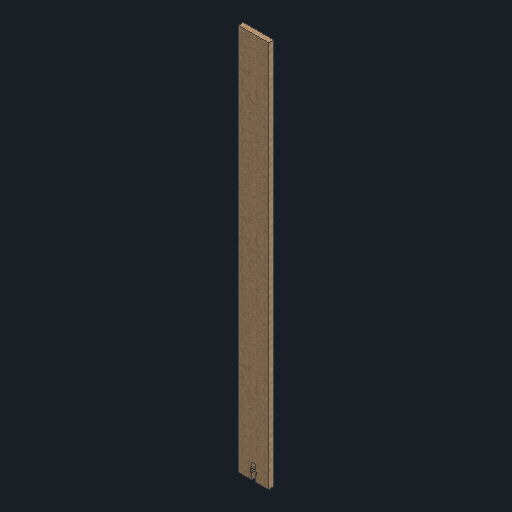
# Autodesk Inventor part: Reed_Rail
Saved by Autodesk Inventor 2024.1 (Build 281209000, 209)
## iProperties
Created: 2023-08-05
Part Number: Reed_Rail
Material: MDF Medium Density Fiberboard
Document SubType Name: Modeling
Designer: jaege
Density: 0.8 g/cm^3
Appearance: Cardboard - Corrugated
Author: jaege
Autodesk Inventor part; units mm, degrees
ref_plane "YZ Plane" through (0, 0, 0) normal (1, 0, 0) x (0, 1, 0)
ref_plane "XZ Plane" through (0, 0, 0) normal (0, 1, 0) x (-1, 0, 0)
ref_plane "XY Plane" through (0, 0, 0) normal (0, 0, 1) x (1, 0, 0)
sketch "Sketch1" plane through (0, 0, 0) normal (0, 0, 1) x (1, 0, 0)
  line L0 (-7, 315) -> (1, 315) projected
  line L1 (-7, 311) -> (-7, 315) projected
  line L2 (1, 311) -> (-7, 311) projected
  line L3 (1, 311) -> (1, 315) projected
  line L4 (-15, 311) -> (9, 311)
  line L5 (9, 311) -> (9, 4)
  line L6 (9, 4) -> (-15, 4)
  line L7 (-15, 4) -> (-15, 311)
  line L8 (-4.5, 4) -> (-1.5, 4)
  line L9 (-1.5, 4) -> (-1.5, 16)
  line L10 (-1.5, 16) -> (-4.5, 16)
  line L11 (-4.5, 16) -> (-4.5, 4)
  line L12 (-5.7, 11.2) -> (-0.3, 11.2)
  line L13 (-0.3, 11.2) -> (-0.3, 8.8)
  line L14 (-0.3, 8.8) -> (-5.7, 8.8)
  line L15 (-5.7, 8.8) -> (-5.7, 11.2)
  point P0 (-3, 311)
  point P1 (-3, 311)
  point P2 (-3, 4)
  point P3 (-3, 4)
  point P4 (-5.7, 10)
  point P5 (-4.5, 10)
  point P6 (-3, 11.2)
  point P7 (-3, 16)
  point P8 (-17.1455, 4)
  point P9 (-4.5, 8.8)
  point P10 (-4.5, 11.2)
  point P11 (-1.5, 11.2)
  point P12 (-1.5, 8.8)
  dimension "d0" = 8
  dimension "d1" = 2.4
  dimension "d2" = 5.4
  dimension "d3" = 3
  dimension "d4" = 12
  constraints: 24 end point, 7 midpoint, 6 parallel, 3 horizontal, 3 horizontal alignment, 3 perpendicular, 2 coincident, 2 vertical alignment, 1 point on line, 1 other
  measures "d0" distance from line of L0.start L7
  measures "d1" distance of L14.end L12.start
  measures "d2" distance of L12.start L12.end
  measures "d3" distance between parallel lines of L9 L11
  measures "d4" distance of L8.end L9.end
extrude "Extrusion1" add sketch "Sketch1" along normal blind 4 contours L2 L4 L5 L6 L9 L14 L13 L12 L10 L11 L15 L7
body "Solid1"
